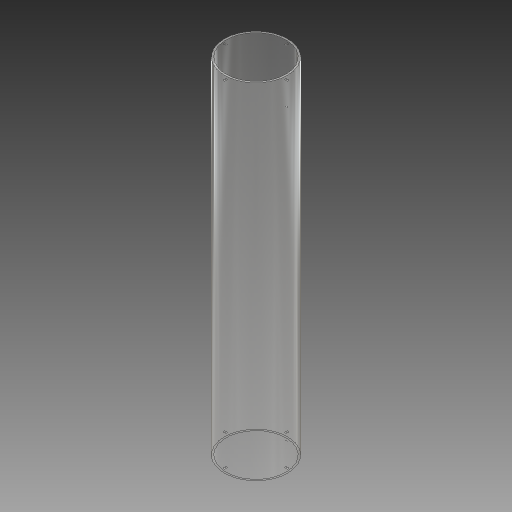
# Autodesk Inventor part: Secondary
Saved by Autodesk Inventor 2019 (Build 230136000, 136)
## iProperties
Created: 2018-04-27
Part Number: Secondary
Material: Polycarbonate, Clear
Document SubType Name: Modeling
Designer: Phil Erle
Density: 1.2 g/cm^3
Appearance: Polycarbonate - Clear
Author: Phil Erle
Autodesk Inventor part; units mm, degrees
ref_plane "YZ Plane" through (0, 0, 0) normal (1, 0, 0) x (0, 1, 0)
ref_plane "XZ Plane" through (0, 0, 0) normal (0, 1, 0) x (-1, 0, 0)
ref_plane "XY Plane" through (0, 0, 0) normal (0, 0, 1) x (1, 0, 0)
sketch "Sketch1" plane through (0, 0, 0) normal (0, 0, 1) x (1, 0, 0)
  circle A0 centre (0, 0) radius 52
  circle A1 centre (0, 0) radius 55
  dimension "d0" = 110
  dimension "d1" = 104
  constraints: 2 centre point, 2 coincident
  measures "d0" diameter of A1
  measures "d1" diameter of A0
extrude "Extrusion1" add sketch "Sketch1" along normal blind 600
sketch "Sketch2" plane through (0, 0, 0) normal (1, 0, 0) x (0, 1, 0)
  circle A0 centre (0, 7.5) radius 1.6
  circle A1 centre (0, 592.5) radius 1.6
  line L0 (-55, 0) -> (55, 0) projected
  line L1 (55, 600) -> (-55, 600) projected
  point P0 (0, 0)
  dimension "d4" = 3.2
  dimension "d5" = 3.2
  dimension "d6" = 7.5
  dimension "d7" = 7.5
  constraints: 2 centre point, 2 vertical alignment
  measures "d4" diameter of A0
  measures "d5" diameter of A1
  measures "d6" distance from line of L0 A0.centre
  measures "d7" distance from line of L1 A1.centre
extrude "Extrusion2" cut sketch "Sketch2" along normal through all both and the other way through all
sketch "Sketch3" plane through (0, 0, 0) normal (0, 1, 0) x (-1, 0, 0)
  circle A0 centre (0, 7.5) radius 1.6
  line L0 (-55, 0) -> (55, 0) projected
  circle A1 centre (0, 592.5) radius 1.6
  line L1 (55, 600) -> (-55, 600) projected
  point P0 (0, 0)
  point P1 (0, 0)
  dimension "d10" = 3.2
  dimension "d11" = 7.5
  dimension "d12" = 3.2
  dimension "d13" = 7.5
  constraints: 2 centre point, 2 vertical alignment, 1 midpoint
  measures "d10" diameter of A0
  measures "d11" distance from line of L0 A0.centre
  measures "d12" diameter of A1
  measures "d13" distance from line of L1 A1.centre
extrude "Extrusion3" cut sketch "Sketch3" along normal through all both and the other way through all
sketch "Sketch4" plane through (0, 0, 0) normal (1, 0, 0) x (0, 1, 0)
  circle A0 centre (0, 48) radius 0.5
  circle A1 centre (0, 552) radius 0.5
  line L0 (-55, 0) -> (55, 0) projected
  line L1 (55, 600) -> (-55, 600) projected
  point P0 (0, 0)
  point P1 (0, 0)
  dimension "d16" = 1
  dimension "d17" = 1
  dimension "d18" = 48
  dimension "d19" = 48
  constraints: 2 centre point, 2 vertical alignment, 1 midpoint
  measures "d16" diameter of A0
  measures "d17" diameter of A1
  measures "d18" distance from line of L0 A0.centre
  measures "d19" distance from line of L1 A1.centre
extrude "Extrusion4" cut sketch "Sketch4" along normal through all
body "Solid1"
